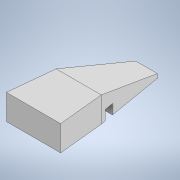
# Autodesk Inventor part: FP Front Hood
Saved by Autodesk Inventor 2020 (Build 240168000, 168)
## iProperties
Created: 2021-04-23
Part Number: FP Front Hood
Material: Generic
Document SubType Name: Modeling
Designer: austi
Density: 1 g/cm^3
Appearance: Default
Author: austi
Autodesk Inventor part; units mm, degrees
ref_plane "YZ Plane" through (0, 0, 0) normal (1, 0, 0) x (0, 1, 0)
ref_plane "XZ Plane" through (0, 0, 0) normal (0, 1, 0) x (-1, 0, 0)
ref_plane "XY Plane" through (0, 0, 0) normal (0, 0, 1) x (1, 0, 0)
sketch "Sketch1" plane through (0, 0, 0) normal (0, 1, 0) x (-1, 0, 0)
  line L0 (15, 25) -> (-15, 25)
  line L1 (12.5, 0) -> (-12.5, 0)
  line L2 (6, -37.5) -> (-6, -37.5)
  line L3 (15, 25) -> (12.5, 0)
  line L4 (6, -37.5) -> (12.5, 0)
  line L5 (-15, 25) -> (-12.5, 0)
  line L6 (-12.5, 0) -> (-6, -37.5)
  line L7 (21, 0) -> (-21, 0) projected
  line L8 (0, -50) -> (0, 37.5) projected
  point P0 (0, 0)
  point P1 (0, 25)
  point P2 (0, 0)
  point P3 (0, -37.5)
  dimension "d0" = 30
  dimension "d1" = 25
  dimension "d2" = 12
  dimension "d3" = 25
  dimension "d4" = 37.5
  constraints: 14 end point, 3 horizontal, 3 midpoint, 2 coincident, 2 vertical alignment, 2 other
  measures "d0" distance of L0.start L0.end
  measures "d1" distance of L1.start L1.end
  measures "d2" distance of L2.start L2.end
  measures "d3" distance between parallel lines of L1 L0
  measures "d4" distance between parallel lines of L2 L1
extrude "Extrusion1" add sketch "Sketch1" along normal blind 14 contours L3 L1 L8 L0 | L8 L1 L5 L0
sketch "Sketch2" plane through (0, 0, 0) normal (0, 1, 0) x (-1, 0, 0)
  line L0 (6, -37.5) -> (-6, -37.5)
  line L1 (-12.5, 0) -> (12.5, 0) projected
  line L2 (12.5, 0) -> (15, 25) projected
  line L3 (12.5, 0) -> (6, -37.5)
  line L4 (-12.5, 0) -> (-6, -37.5)
  line L5 (12.5, 0) -> (-12.5, 0)
  point P0 (0, 0)
  point P1 (0, -37.5)
  point P2 (0, 0)
  dimension "d7" = 12
  dimension "d8" = 37.5
  constraints: 8 end point, 2 midpoint, 1 collinear, 1 horizontal, 1 vertical alignment
  measures "d7" distance of L0.start L0.end
  measures "d8" distance between parallel lines of L0 L1
extrude "Extrusion2" add sketch "Sketch2" along normal blind 14
sketch "Sketch3" plane through (0, 0, 0) normal (1, 0, 0) x (0, 1, 0)
  line L0 (-2.8, 0) -> (16.8, 0) projected
  line L1 (0, -50) -> (0, 37.5) projected
  line L2 (0, -37.5) -> (14, -37.5) projected
  line L3 (14, -37.5) -> (14, 0) projected
  line L4 (0, -37.5) -> (0, 0) projected
  line L5 (14, 0) -> (14, 25) projected
  line L6 (0, 25) -> (14, 25) projected
  line L7 (0, 0) -> (14, 0) projected
  line L8 (0, -37.5) -> (2.25, -37.5)
  line L9 (2.25, -37.5) -> (14, 0)
  line L10 (14, 0) -> (14, -37.5)
  line L11 (2.25, -37.5) -> (14, -37.5)
  dimension "d11" = 2.25
  constraints: 8 end point, 1 collinear, 1 perpendicular, 1 point on line
  measures "d11" distance of L2.start L8.end
extrude "Extrusion3" cut sketch "Sketch3" along normal through all both and the other way through all contours L3 L2 L9
sketch "Sketch4" plane through (0, 0, 0) normal (0, -1, 0) x (1, 0, 0)
  line L0 (12.5, 0) -> (6, -37.5) projected
  line L1 (12.0667, -2.5) -> (-12.0667, -2.5)
  line L2 (-6, -37.5) -> (-12.5, 0) projected
  line L3 (11.2, -7.5) -> (-11.2, -7.5)
  line L4 (-15, 25) -> (15, 25) projected
  line L5 (12.0667, -2.5) -> (11.2, -7.5)
  line L6 (-12.0667, -2.5) -> (-11.2, -7.5)
  point P0 (0, 0)
  dimension "d14" = 27.5
  dimension "d15" = 5
  constraints: 8 end point, 4 point on line, 2 horizontal, 1 collinear
  measures "d14" distance between parallel lines of L1 L4
  measures "d15" distance between parallel lines of L3 L1
extrude "Extrusion4" cut sketch "Sketch4" against normal blind 5.5
body "Solid1"
